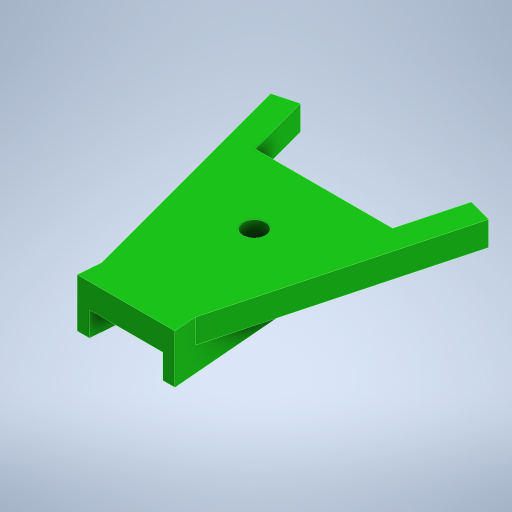
# Autodesk Inventor part: Servo Arm
Saved by Autodesk Inventor 2023 (Build 270158000, 158)
## iProperties
Created: 2022-10-14
Part Number: Servo Arm
Material: Generic
Document SubType Name: Modeling
Designer: GROS
Density: 1 g/cm^3
Appearance: Dark Green
Author: GROS
Autodesk Inventor part; units mm, degrees
ref_plane "YZ Plane" through (0, 0, 0) normal (1, 0, 0) x (0, 1, 0)
ref_plane "XZ Plane" through (0, 0, 0) normal (0, 1, 0) x (-1, 0, 0)
ref_plane "XY Plane" through (0, 0, 0) normal (0, 0, 1) x (1, 0, 0)
sketch "Sketch1" plane through (0, 0, 0) normal (0, 1, 0) x (-1, 0, 0)
  circle A0 centre (0, 0) radius 0.5
  line L0 (0, 0) -> (0, -2)
  circle A1 centre (0, -2) radius 0.75
  line L1 (0, -2) -> (0, -4)
  line L2 (0, -4) -> (0, -6)
  circle A2 centre (0, -4) radius 0.5
  circle A3 centre (0, -6) radius 0.5
  line L3 (0, 1.25) -> (0, 0)
  line L4 (0, 0.5) -> (0, 4.8)
  line L5 (0, 4.8) -> (0, -22.2)
  line L6 (0, -6.5) -> (0, -8)
  line L7 (0, -6) -> (0, -8)
  circle A4 centre (0, -8) radius 0.5
  line L8 (0, -8.5) -> (0, -12.5)
  line L9 (0, -12.5) -> (0, -12)
  circle A5 centre (0, -10.5) radius 0.925
  circle A6 centre (0, -12) radius 0.5
  line L10 (0, 1.25) -> (3, 1.25)
  line L11 (3, 1.25) -> (-3, 1.25)
  line L12 (-3, 1.25) -> (-3, -13.75)
  line L13 (-3, -13.75) -> (3, -13.75)
  line L14 (3, -13.75) -> (3, 1.25)
  line L15 (3, 0) -> (-3, 0)
  line L16 (0, -12) -> (2, -12)
  line L17 (2, -12) -> (-2, -12)
  line L18 (-2, -12) -> (-3, 0)
  line L19 (2, -12) -> (3, 0)
  line L20 (3, 0) -> (4, 0)
  line L21 (2, -12) -> (3, -12)
  line L22 (3, -12) -> (4, 0)
  line L23 (-3, 0) -> (-4, 0)
  line L24 (-2, -12) -> (-3, -12)
  line L25 (-4, 0) -> (-3, -12)
  line L26 (0, 4.8) -> (6.9881, -21.28)
  line L27 (0, 4.8) -> (-6.9881, -21.28)
  line L28 (-6.9881, -21.28) -> (-8.9881, -21.28)
  line L29 (-6.9881, -21.28) -> (-8.92, -20.7624)
  line L30 (-8.92, -20.7624) -> (-8.92, -1.1218)
  line L31 (-8.92, -20.7624) -> (-3.8366, -1.791)
  line L32 (6.9881, -21.28) -> (8.9881, -21.28)
  line L33 (6.9881, -21.28) -> (8.92, -20.7624)
  line L34 (8.92, -20.7624) -> (8.92, -0.4933)
  line L35 (8.92, -20.7624) -> (3.674, -1.184)
  line L36 (0, -22.2) -> (0, -16.2)
  line L37 (0, -16.2) -> (5.6269, -16.2)
  line L38 (0, -16.2) -> (-5.6269, -16.2)
  point P0 (0, -11.5)
  point P1 (3.8474, -1.8313)
  point P2 (-3.8474, -1.8313)
  dimension "d0" = 1
  dimension "d6" = 1
  dimension "d42" = 1
  dimension "d1" = 2
  dimension "d2" = 1.5
  dimension "d3" = 2
  dimension "d4" = 2
  dimension "d5" = 1
  dimension "d10" = 1.25
  dimension "d13" = 4.3
  dimension "d16" = 27
  dimension "d41" = 2
  dimension "d43" = 4
  dimension "d44" = 0.5
  dimension "d45" = 1
  dimension "d46" = 1.85
  dimension "d47" = 3
  dimension "d48" = 6
  dimension "d49" = 15
  dimension "d61" = 2
  dimension "d62" = 4
  dimension "d63" = 1
  dimension "d64" = 1
  dimension "d65" = 1
  dimension "d66" = 1
  dimension "d69" = 2
  dimension "d70" = 27
  dimension "d71" = 27
  dimension "d72" = 2
  dimension "d73" = 2
  dimension "d75" = 2
  dimension "d76" = 2
  dimension "d77" = 6
  constraints: 78 end point, 12 point on line, 9 horizontal, 6 coincident, 4 centre point, 3 vertical alignment, 2 parallel, 2 perpendicular, 2 vertical, 1 midpoint, 6 other
  measures "d1" distance of L0.start L0.end
  measures "d2" diameter of A1
  measures "d3" distance of L1.start L1.end
  measures "d4" distance of L1.end L2.end
  measures "d5" diameter of A2
  measures "d10" distance of L3.start L0.start
  measures "d13" distance of L4.start L4.end
  measures "d16" distance of L4.end L5.end
  measures "d41" distance of L7.start L7.end
  measures "d43" distance of L8.end L8.start
  measures "d44" distance of L9.end point (0, -11.5)
  measures "d45" diameter of A6
  measures "d46" diameter of A5
  measures "d47" distance of L3.start L10.end
  measures "d48" distance of L10.end L11.end
  measures "d49" distance of L13.end L10.end
  measures "d61" distance of L16.start L16.end
  measures "d62" distance of L16.end L17.end
  measures "d63" distance of L15.start L20.end
  measures "d64" distance of L16.end L21.end
  measures "d65" distance of L17.end L24.end
  measures "d66" distance of L15.end L23.end
  measures "d69" distance of A5.centre L8.start
  measures "d70" distance of L26.start L26.end
  measures "d71" distance of L27.start L27.end
  measures "d72" distance of L27.end L28.end
  measures "d73" distance of L29.start L29.end
  measures "d75" distance of L26.end L32.end
  measures "d76" distance of L33.start L33.end
  measures "d77" distance of L5.end L36.end
extrude "Extrusion1" add sketch "Sketch1" along normal blind 2 contours L15 L26 L19 L16 A6 L5 A5 A4 A3 L2 A2 L1 A1 L0 A0 | A0 L0 L15 | L0 A1 L1 A2 L2 A3 L5 A4 A5 A6 L17 L18 L27 L15 A0 | A0 L15 L0 | L15 L19 L26 | A1 L1 L0 | L0 L1 A1 | L20 L22 L26 L14 | L14 L26 L19 | L26 L14 L21 L19 | L27 L18 L15 | L26 L22 L14 | L21 L14 L13 L5 A6 L16 | L18 L27 L12 | L12 L27 L25 L23 | L18 L24 L12 L27 | A2 L2 L1 | L1 L2 A2 | L22 L26 L37 L5 L13 L14 | L22 L35 L33 L26 | L16 L5 A6 | A6 L5 L16 | L12 L25 L27 | L17 A6 L5 L13 L12 L24 | A6 L17 L5 | L5 L17 A6 | L12 L13 L5 L38 L27 L25 | L27 L29 L31 L25 | A3 L5 L2 | L2 L5 A3 | A4 L5 | L5 A4
extrude "Extrusion2" add sketch "Sketch1" against normal blind 2 contours L20 L22 L26 L14 | L14 L26 L19 | L26 L14 L21 L19 | L26 L22 L14 | L18 L27 L12 | L12 L27 L25 L23 | L18 L24 L12 L27 | L12 L25 L27
body "Solid1"
